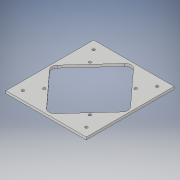
# Autodesk Inventor part: 板子3
Saved by Autodesk Inventor 2017 (Build 210142000, 142)
## iProperties
Part Number: 板子3
Material: 一般
Document SubType Name: Modeling
Designer: User
Density: 1 g/cm^3
Appearance: 預設
Author: User
Autodesk Inventor part; units mm, degrees
ref_plane "YZ Plane" through (0, 0, 0) normal (1, 0, 0) x (0, 1, 0)
ref_plane "XZ Plane" through (0, 0, 0) normal (0, 1, 0) x (-1, 0, 0)
ref_plane "XY Plane" through (0, 0, 0) normal (0, 0, 1) x (1, 0, 0)
sketch "草圖1" plane through (0, 0, 0) normal (0, 1, 0) x (-1, 0, 0)
  line L0 (47.5, 51.85) -> (-47.5, 51.85)
  line L1 (-47.5, 51.85) -> (-47.5, -51.85)
  line L2 (-47.5, -51.85) -> (47.5, -51.85)
  line L3 (47.5, -51.85) -> (47.5, 51.85)
  line L4 (43.1682, 4.7285) -> (5.1615, 46.2158)
  line L5 (-43.1682, 4.7285) -> (-5.1615, 46.2158)
  line L6 (43.1682, -4.7285) -> (5.1615, -46.2158)
  line L7 (-43.1682, -4.7285) -> (-5.1615, -46.2158)
  arc A0 (43.1682, -4.7285) -> (43.1682, 4.7285) centre (38.0067, 0) ccw
  arc A1 (-5.1615, -46.2158) -> (5.1615, -46.2158) centre (0, -41.4873) ccw
  arc A2 (-43.1682, 4.7285) -> (-43.1682, -4.7285) centre (-38.0067, 0) ccw
  arc A3 (5.1615, 46.2158) -> (-5.1615, 46.2158) centre (0, 41.4873) ccw
  line L8 (47.5, -51.85) -> (47.5, -41.85)
  circle A4 centre (37.5, -41.85) radius 1.5
  circle A5 centre (27, -27) radius 1.5
  circle A6 centre (-27, 27) radius 1.5
  circle A7 centre (-37.5, 41.85) radius 1.5
  line L9 (66.5, 0) -> (-66.5, 0) projected
  circle A8 centre (37.5, 41.85) radius 1.5
  circle A9 centre (27, 27) radius 1.5
  circle A10 centre (-27, -27) radius 1.5
  circle A11 centre (-37.5, -41.85) radius 1.5
  line L10 (27, -27) -> (0, 0)
  line L11 (0, 0) -> (30, 0)
  line L12 (30, 0) -> (30, -30)
  line L13 (30, -30) -> (0, -30)
  line L14 (0, -30) -> (0, 0)
  point P0 (47.5, 0)
  point P1 (0, 51.85)
  point P2 (-47.5, 0)
  point P3 (0, -51.85)
  dimension "d88" = 103.7
  dimension "d89" = 95
  dimension "d90" = 47.5
  dimension "d91" = 51.85
  dimension "d92" = 7
  dimension "d95" = 3
  dimension "d98" = 3
  dimension "d101" = 360
  dimension "d103" = 30
  dimension "d104" = 30
  dimension "d105" = 3
  dimension "d106" = 3
  constraints: 28 end point, 12 centre point, 9 point on line, 8 point on circle, 8 tangent, 5 parallel, 4 midpoint, 4 symmetric about line, 3 equal radius, 2 horizontal, 2 perpendicular, 13 other
  measures "d88" distance of L2.end L0.start
  measures "d89" distance of L1.end L2.end
  measures "d90" distance from line of L10.end L3
  measures "d91" distance from line of L10.end L2
  measures "d92" radius of A0
  measures "d95" diameter of A4
  measures "d98" diameter of A5
  measures "d103" distance of L11.end L12.end
  measures "d104" distance of L12.end L13.end
  measures "d105" distance from line of L10.start L12
  measures "d106" distance from line of L13 L10.start
extrude "擠出2" add sketch "草圖1" along normal mid plane 3 contours L3 L9 A0 L4 A3 L5 A2 L1 L0 | L3 L2 L1 L9 A2 L7 A1 L6 L13 L12 A0 | L12 L13 L6
